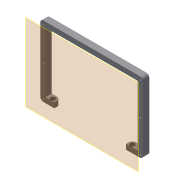
# Autodesk Inventor part: cellSTORM_v5_electronicbox
Saved by Autodesk Inventor 2019.4 (Build 234330000, 330)
## iProperties
Created: 2021-08-24
Part Number: cellSTORM_v5_electronicbox
Material: Generic
Document SubType Name: Modeling
Designer: diederichbenedict
Density: 1 g/cm^3
Appearance: Default
Author: diederichbenedict
Autodesk Inventor part; units mm, degrees
ref_plane "YZ Plane" through (0, 0, 0) normal (1, 0, 0) x (0, 1, 0)
ref_plane "XZ Plane" through (0, 0, 0) normal (0, 1, 0) x (-1, 0, 0)
ref_plane "XY Plane" through (0, 0, 0) normal (0, 0, 1) x (1, 0, 0)
ref_plane "Work Plane1" through (0, 0, 25) normal (0, 0, 1) x (1, 0, 0)
sketch "Sketch1" plane through (0, 0, 25) normal (0, 0, 1) x (1, 0, 0)
  circle A0 centre (38.8114, -42.6244) radius 3.5 projected
  circle A1 centre (38.8114, -18.3756) radius 3.5 projected
  circle A2 centre (59.8114, -30.5) radius 3.5 projected
  circle A3 centre (-41, 0) radius 4 projected
  circle A4 centre (9, 0) radius 4 projected
  circle A5 centre (-41, 50) radius 4 projected
  circle A6 centre (-16, 50) radius 4 projected
  circle A7 centre (9, 25) radius 4 projected
  circle A8 centre (-16, 0) radius 4 projected
  circle A9 centre (-41, 25) radius 4 projected
  line L0 (4, 5) -> (4, 45) projected
  line L1 (-36, 5) -> (4, 5) projected
  line L2 (-36, 45) -> (-36, 5) projected
  line L3 (4, 45) -> (-36, 45) projected
  line L4 (-75, 55) -> (75, 55) projected
  line L5 (-80, -50) -> (-80, 50) projected
  line L6 (75, -55) -> (-75, -55) projected
  line L7 (80, 50) -> (80, -50) projected
  arc A10 (80, 50) -> (75, 55) centre (75, 50) ccw projected
  arc A11 (-75, 55) -> (-80, 50) centre (-75, 50) ccw projected
  arc A12 (-80, -50) -> (-75, -55) centre (-75, -50) ccw projected
  arc A13 (75, -55) -> (80, -50) centre (75, -50) ccw projected
  arc A14 (5.1102, 49.0673) -> (5.3508, 51.638) centre (9, 50) ccw projected
  arc A15 (2.6606, 50.5554) -> (5.1102, 49.0673) centre (4, 50) ccw projected
  arc A16 (5.3508, 51.638) -> (2.6606, 50.5554) centre (4, 51.1109) ccw projected
  circle A17 centre (-76, 50) radius 1.45 projected
  circle A18 centre (-75.7071, -50.7071) radius 1.45 projected
  circle A19 centre (76, 0) radius 1.45 projected
  circle A20 centre (75.7071, 50.7071) radius 1.45 projected
  circle A21 centre (75.7071, -50.7071) radius 1.45 projected
  circle A22 centre (4, -51) radius 1.45 projected
  circle A23 centre (-76, -2.5) radius 1.45 projected
  point P0 (0, 0)
extrude "Extrusion1" add sketch "Sketch1" along normal blind 5 contours A0 | A1 | A2 | A3 | A4 | A5 | A6 | A7 | A8 | A9 | L1 L2 L3 L0 | L4 A10 L7 A13 L6 A12 L5 A11 | A15 A16 A14 | A17 | A18 | A19 | A20 | A21 | A22 | A23
sketch "Sketch2" plane through (0, 0, 30) normal (0, 0, 1) x (-1, 0, 0)
  line L0 (-75, -55) -> (75, -55) projected
  line L1 (-80, 50) -> (-80, -50) projected
  line L2 (75, 55) -> (-75, 55) projected
  line L3 (80, -50) -> (80, 50) projected
  line L4 (75, -55) -> (-75, -55) projected
  line L5 (-80, -50) -> (-80, 50) projected
  line L6 (-75, 55) -> (75, 55) projected
  line L7 (80, 50) -> (80, -50) projected
  line L8 (-72, 47) -> (-72, -47)
  line L9 (-72, -47) -> (72, -47)
  line L10 (72, -47) -> (72, 47)
  line L11 (72, 47) -> (-72, 47)
  arc A0 (-80, -50) -> (-75, -55) centre (-75, -50) ccw projected
  arc A1 (-75, 55) -> (-80, 50) centre (-75, 50) ccw projected
  arc A2 (80, 50) -> (75, 55) centre (75, 50) ccw projected
  arc A3 (75, -55) -> (80, -50) centre (75, -50) ccw projected
  arc A4 (75, -55) -> (80, -50) centre (75, -50) ccw projected
  arc A5 (80, 50) -> (75, 55) centre (75, 50) ccw projected
  arc A6 (-75, 55) -> (-80, 50) centre (-75, 50) ccw projected
  arc A7 (-80, -50) -> (-75, -55) centre (-75, -50) ccw projected
  dimension "d8" = 8
  constraints: 8 end point, 3 other
  measures "d8" distance between parallel lines of L2 L11
ref_plane "Work Plane2" through (-80, -55, 0) normal (0, 0, 1) x (1, 0, 0)
extrude "Extrusion2" add sketch "Sketch2" against normal up to surface (30 mm away)
sketch "Sketch3" plane through (-80, -55, 25) normal (0, -1, 0) x (1, 0, 0)
  line L0 (152, -5) -> (152, -25) projected
  line L1 (8, -5) -> (8, -25) projected
  line L2 (8, -5) -> (8, -25) projected
  line L3 (152, -25) -> (8, -25)
  line L4 (8, -25) -> (8, -5)
  line L5 (8, -5) -> (152, -5)
  line L6 (152, -5) -> (152, -25)
  line L7 (8, -5) -> (152, -5) projected
  line L8 (5, 5) -> (155, 5) projected
  line L9 (133.7332, -5) -> (21.8933, -5)
  line L10 (21.8933, -5) -> (21.8933, -55.1362)
  line L11 (21.8933, -55.1362) -> (133.7332, -55.1362)
  line L12 (133.7332, -55.1362) -> (133.7332, -5)
  line L13 (133.7332, -5) -> (21.8933, -55.1362) construction
  line L14 (21.8933, -5) -> (133.7332, -55.1362) construction
  line L15 (155, -25) -> (5, -25) projected
  line L16 (155, 5) -> (155, -25) projected
  line L17 (5, 5) -> (5, -25) projected
  point P0 (77.8132, -30.0681)
  dimension "d9" = 0
  constraints: 20 end point, 4 parallel, 2 horizontal, 2 midpoint, 2 perpendicular
  measures "d9" distance between parallel lines of L5 L9
extrude "Extrusion3" cut sketch "Sketch3" against normal blind 10 contours L12 L3 L10 L5 | L12 L11 L10 L3
fillet "Fillet1" radius 6 4 edges at (53.7332, -51, 0) (53.7332, -51, 20) (-58.1067, -51, 20) (-58.1067, -51, 0)
fillet "Fillet2" radius 6 4 edges at (80, 0, 30) (0, -55, 30) (-80, 0, 30) (0, 55, 30)
sketch "Sketch4" plane through (75, 55, 0) normal (0, 0, -1) x (-1, 0, 0)
  line L0 (139.1067, -110) -> (139.1067, -102) projected
  line L1 (139.1067, -110) -> (150, -110) projected
  arc A0 (150, -110) -> (155, -105) centre (150, -105) ccw projected
  line L2 (155, -105) -> (155, -5) projected
  arc A1 (155, -5) -> (150, 0) centre (150, -5) ccw projected
  line L3 (150, 0) -> (0, 0) projected
  arc A2 (0, 0) -> (-5, -5) centre (0, -5) ccw projected
  line L4 (-5, -5) -> (-5, -105) projected
  arc A3 (-5, -105) -> (0, -110) centre (0, -105) ccw projected
  line L5 (0, -110) -> (15.2668, -110) projected
  line L6 (15.2668, -102) -> (15.2668, -110) projected
  line L7 (15.2668, -102) -> (3, -102) projected
  line L8 (3, -102) -> (3, -8) projected
  line L9 (3, -8) -> (147, -8) projected
  line L10 (147, -8) -> (147, -102) projected
  line L11 (147, -102) -> (139.1067, -102) projected
  arc A4 (0, 0) -> (-5, -5) centre (0, -5) ccw projected
  line L12 (150, 0) -> (0, 0) projected
  arc A5 (155, -5) -> (150, 0) centre (150, -5) ccw projected
  line L13 (155, -105) -> (155, -5) projected
  arc A6 (150, -110) -> (155, -105) centre (150, -105) ccw projected
  line L14 (0, -110) -> (150, -110) projected
  arc A7 (-5, -105) -> (0, -110) centre (0, -105) ccw projected
  line L15 (-5, -5) -> (-5, -105) projected
  circle A8 centre (36.1886, -97.6244) radius 3.5 projected
  circle A9 centre (36.1886, -73.3756) radius 3.5 projected
  circle A10 centre (15.1886, -85.5) radius 3.5 projected
  circle A11 centre (116, -55) radius 4 projected
  circle A12 centre (66, -55) radius 4 projected
  arc A13 (69.8897, -5.9327) -> (72.3394, -4.4446) centre (71, -5) ccw projected
  arc A14 (72.3394, -4.4446) -> (69.6492, -3.362) centre (71, -3.8891) ccw projected
  arc A15 (69.6492, -3.362) -> (69.8897, -5.9327) centre (66, -5) ccw projected
  circle A16 centre (116, -5) radius 4 projected
  circle A17 centre (91, -5) radius 4 projected
  circle A18 centre (66, -30) radius 4 projected
  circle A19 centre (91, -55) radius 4 projected
  circle A20 centre (116, -30) radius 4 projected
  line L16 (71, -50) -> (71, -10) projected
  line L17 (111, -50) -> (71, -50) projected
  line L18 (111, -10) -> (111, -50) projected
  line L19 (71, -10) -> (111, -10) projected
  circle A21 centre (151, -5) radius 1.45 projected
  circle A22 centre (150.7071, -105.7071) radius 1.45 projected
  circle A23 centre (-1, -55) radius 1.45 projected
  circle A24 centre (-0.7071, -4.2929) radius 1.45 projected
  circle A25 centre (-0.7071, -105.7071) radius 1.45 projected
  circle A26 centre (71, -106) radius 1.45 projected
  circle A27 centre (151, -57.5) radius 1.45 projected
  point P0 (75, -55)
hole "Hole1" at (75.7071, -50.7071, 0) at (76, 0, 0) at (75.7071, 50.7071, 0) at (-75.7071, -50.7071, 0) at (-76, -2.5, 0) at (-76, 50, 0) direction (0, 0, 1) diameter 2.9 depth 15 tip angle 118
sketch "Sketch5" plane through (0, 0, 30) normal (0, 0, 1) x (1, 0, 0)
  line L0 (-60, 40) -> (60, 40)
  line L1 (60, 40) -> (60, -40)
  line L2 (60, -40) -> (-60, -40)
  line L3 (-60, -40) -> (-60, 40)
  line L4 (-60, 40) -> (60, -40) construction
  line L5 (60, 40) -> (-60, -40) construction
  circle A0 centre (60, -40) radius 1.45
  point P0 (0, 0)
  dimension "d19" = 120
  dimension "d20" = 80
  dimension "d21" = 2.9
  constraints: 12 end point, 2 midpoint, 2 parallel, 1 centre point, 1 coincident, 1 horizontal, 1 perpendicular
  measures "d19" distance of L1.end L2.end
  measures "d20" distance of L0.end L1.end
  measures "d21" diameter of A0
extrude "Extrusion4" cut sketch "Sketch5" against normal blind 10 contours A0 L2 L1 | L1 L2 A0
pattern_linear "Rectangular Pattern1" count 7 spacing 20 along (-1, 0, 0) count 5 spacing 20 along (0, 1, 0) of "Extrusion4"
sketch "Sketch6" plane through (-72, -47, 25) normal (0, 1, 0) x (1, 0, 0)
  arc A0 (13.8933, 19) -> (7.8933, 25) centre (7.8933, 19) ccw projected
  arc A1 (131.7332, 25) -> (125.7332, 19) centre (131.7332, 19) ccw projected
  circle A2 centre (7.8933, 19) radius 4
  circle A3 centre (131.7332, 19) radius 4
  point P0 (72, 25)
  dimension "d30" = 8
  dimension "d31" = 8
  constraints: 2 centre point, 2 coincident
  measures "d30" diameter of A2
  measures "d31" diameter of A3
extrude "Extrusion5" cut sketch "Sketch6" against normal blind 7
sketch "Sketch7" plane through (75, 55, 0) normal (0, 0, -1) x (-1, 0, 0)
  line L0 (221.0229, 19.1465) -> (-79.5928, 19.1465)
  line L1 (-79.5928, 19.1465) -> (-79.5928, -151.414)
  line L2 (-79.5928, -151.414) -> (221.0229, -151.414)
  line L3 (221.0229, -151.414) -> (221.0229, 19.1465)
  point P0 (75, -55)
  constraints: 8 end point, 2 parallel, 1 horizontal, 1 perpendicular
extrude "Extrusion6" cut sketch "Sketch7" against normal blind 10 keep common part
body "Solid1"
